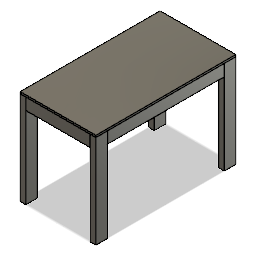
WorkBench v1 (Autodesk Fusion 360 design; units mm, degrees)
Autodesk Fusion 360 part; units mm, degrees
sketch "Sketch1" plane through (0, 0, 0) normal (1, 0, 0) x (0, 0, -1)
  line L0 (0, 0) -> (-101.6, 0)
  line L1 (-101.6, 0) -> (-101.6, 711.2)
  line L2 (-101.6, 711.2) -> (0, 711.2)
  line L3 (0, 711.2) -> (0, 0)
  dimension "d1" = 101.6
  dimension "d2" = 711.2
  constraint horizontal L0
  constraint vertical L1
  constraint horizontal L2
  constraint vertical L3
  constraint coincident L0.start L3.end
  measures "d1" distance of L0.start L0.end
  measures "d2" distance of L0.start L2.end
extrude "Extrude1" add sketch "Sketch1" along normal blind 50.8 makes body 1
sketch "Sketch2" plane through (0, 0, 0) normal (0, 0, -1) x (-1, 0, 0)
  line L0 (0, 0) -> (0, 711.2)
  line L1 (0, 711.2) -> (-50.8, 711.2)
  line L2 (-50.8, 711.2) -> (-50.8, 0)
  line L3 (-50.8, 0) -> (0, 0)
  line L4 (-50.8, 711.2) -> (0, 711.2)
  line L5 (0, 711.2) -> (0, 609.6)
  line L6 (0, 609.6) -> (-50.8, 609.6)
  line L7 (-50.8, 609.6) -> (-50.8, 711.2)
  dimension "d5" = 101.6
  constraint horizontal L4
  constraint vertical L5
  constraint horizontal L6
  constraint vertical L7
  constraint coincident L1.end L2.start
  measures "d5" distance of L1.end L6.end
extrude "Extrude2" add sketch "Sketch2" along normal blind 1016 separate body contours L0 L1 L2 L4 L5 L6 L7 makes body 2
sketch "Sketch3" plane through (0, 711.2, 0) normal (0, 1, 0) x (-1, 0, 0)
  line L0 (0, 0) -> (-50.8, 0)
  line L1 (-50.8, 0) -> (-50.8, -1016)
  line L2 (-50.8, -1016) -> (0, -1016)
  line L3 (0, -1016) -> (0, 0)
  line L4 (0, -1016) -> (-50.8, -1016)
  line L5 (-50.8, -1016) -> (-50.8, -1117.6)
  line L6 (-50.8, -1117.6) -> (0, -1117.6)
  line L7 (0, -1117.6) -> (0, -1016)
  constraint horizontal L4
  constraint vertical L5
  constraint horizontal L6
  constraint vertical L7
  constraint coincident L2.end L3.start
extrude "Extrude3" add sketch "Sketch3" against normal blind 711.2 separate body contours L2 L4 L5 L6 L7 makes body 3
move_body "Move1" bodies 2 to x (1, 0, 0) y (0, 1, 0) z (0, 0, 1) at (0, 101.6, 0)
extrude "Extrude4" add 2 faces at (33.8667, 711.2, 67.7333) (33.8667, 711.2, -1049.8667) along direction (0, 1, 0) blind 101.6 on bodies 1 3 bodies 1 3
copy_body "CopyPasteBodies1" bodies 1 2 3 makes body 4 makes body 5 makes body 6
move_body "Move2" bodies 4 5 6 to x (1, 0, 0) y (0, 1, 0) z (0, 0, 1) at (609.6, 0, 0)
sketch "Sketch4" plane through (0, 812.8, 0) normal (0, 1, 0) x (-1, 0, 0)
  line L0 (-609.6, -1117.6) -> (-609.6, -1016)
  line L1 (-609.6, -1016) -> (-660.4, -1016)
  line L2 (-660.4, -1016) -> (-660.4, -1117.6)
  line L3 (-660.4, -1117.6) -> (-609.6, -1117.6)
  line L4 (-660.4, -1117.6) -> (0, -1117.6)
  line L5 (0, -1117.6) -> (0, 101.6)
  line L6 (0, 101.6) -> (-660.4, 101.6)
  line L7 (-660.4, 101.6) -> (-660.4, -1117.6)
  point P0 (0, 101.6)
  constraint horizontal L4
  constraint vertical L5
  constraint horizontal L6
  constraint vertical L7
  constraint coincident P0 L5.end
  constraint coincident L2.end L3.start
extrude "Extrude5" add sketch "Sketch4" along normal blind 15.875 separate body makes body 7
sketch "Sketch5" plane through (0, 711.2, 0) normal (0, -1, 0) x (1, 0, 0)
  line L0 (50.8, 0) -> (0, 0)
  line L1 (0, 0) -> (0, -1016)
  line L2 (0, -1016) -> (50.8, -1016)
  line L3 (50.8, -1016) -> (50.8, 0)
  line L4 (50.8, -508) -> (50.8, -482.6)
  line L5 (50.8, -508) -> (50.8, -508)
  line L6 (50.8, -508) -> (50.8, -533.4)
  line L7 (50.8, -533.4) -> (50.8, -533.4)
  line L8 (50.8, -533.4) -> (50.8, -508)
  line L9 (50.8, -533.4) -> (609.6, -533.4)
  line L10 (609.6, -533.4) -> (609.6, -482.6)
  line L11 (609.6, -482.6) -> (50.8, -482.6)
  line L12 (50.8, -482.6) -> (50.8, -533.4)
  dimension "d14" = 25.4
  dimension "d15" = 50.8
  constraint midpoint L3 L4.start
  constraint vertical L6
  constraint vertical L8
  constraint horizontal L9
  constraint vertical L10
  constraint horizontal L11
  constraint vertical L12
  measures "d14" distance of L4.start L4.end
  measures "d15" distance of L6.end L4.end
extrude "Extrude6" add sketch "Sketch5" against normal blind 101.6 separate body contours L3 L4 L6 L8 L9 L10 L11 L12 makes body 8
copy_body "CopyPasteBodies2" bodies 8 makes body 9
move_body "Move3" bodies 9 to x (1, 0, 0) y (0, 1, 0) z (0, 0, 1) at (0, 0, -584.2)
copy_body "CopyPasteBodies3" bodies 8 makes body 10
move_body "Move4" bodies 10 to x (1, 0, 0) y (0, 1, 0) z (0, 0, 1) at (0, 0, 584.2)
equation "d12 = ( 5 / 8 ) * 1 in"
